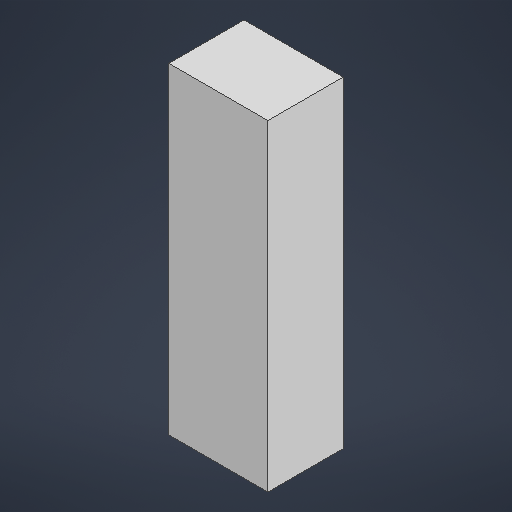
# Autodesk Inventor part: 3sLiPo
Saved by Autodesk Inventor 2026.1 (Build 301233020, 233B)
## iProperties
Created: 2026-03-17
Part Number: 3sLiPo
Material: 一般
Document SubType Name: Modeling
Designer: kamada
Density: 1 g/cm^3
Appearance: 既定
Author: kamada
Autodesk Inventor part; units mm, degrees
ref_plane "YZ Plane" through (0, 0, 0) normal (1, 0, 0) x (0, 1, 0)
ref_plane "XZ Plane" through (0, 0, 0) normal (0, 1, 0) x (-1, 0, 0)
ref_plane "XY Plane" through (0, 0, 0) normal (0, 0, 1) x (1, 0, 0)
sketch "スケッチ1" plane through (0, 0, 0) normal (0, 0, 1) x (1, 0, 0)
  line L0 (-12.9, 41.9) -> (12.9, 41.9)
  line L1 (12.9, 41.9) -> (12.9, -41.9)
  line L2 (12.9, -41.9) -> (-12.9, -41.9)
  line L3 (-12.9, -41.9) -> (-12.9, 41.9)
  point P0 (0, 0)
  point P1 (0, 41.9)
  point P2 (12.9, 0)
  dimension "d0" = 25.8
  dimension "d1" = 83.8
  constraints: 8 end point, 2 midpoint, 2 parallel, 1 horizontal, 1 horizontal alignment, 1 perpendicular, 1 vertical alignment
  measures "d0" distance of L1.end L2.end
  measures "d1" distance of L0.end L1.end
extrude "押し出し1" add sketch "スケッチ1" along normal blind 19.6
